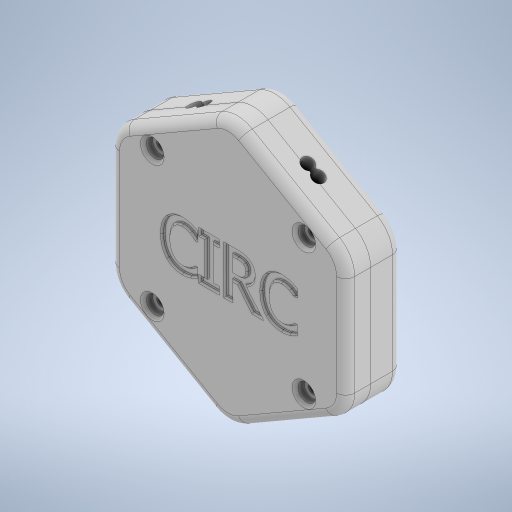
# Autodesk Inventor part: 4-panel splitter
Saved by Autodesk Inventor 2024 (Build 280153020, 153B)
## iProperties
Created: 2023-08-06
Part Number: 4-panel splitter
Material: Generic
Document SubType Name: Modeling
Designer: torban
Density: 1 g/cm^3
Appearance: Default
Author: torban
Autodesk Inventor part; units mm, degrees
(part 1 of 2)
sketch "Sketch2" plane through (0, 0, 0) normal (0, 0, 1) x (1, 0, 0)
  line L0 (0, 0) -> (-18.7, 0)
  line L1 (-18.7, 0) -> (-18.7, 30.4)
  line L2 (-18.7, 30.4) -> (0, 30.4)
  line L3 (0, 30.4) -> (0, 0)
  line L4 (30, 0) -> (48.7, 0)
  line L5 (48.7, 0) -> (48.7, 30.4)
  line L6 (48.7, 30.4) -> (30, 30.4)
  line L7 (30, 30.4) -> (30, 0)
  dimension "d0" = 18.7
  dimension "d1" = 30.4
  dimension "d2" = 30
  dimension "d3" = 30.4
  dimension "d4" = 18.7
  dimension "d5" = 30.4
  constraints: 16 end point, 4 parallel, 2 horizontal, 2 perpendicular
  measures "d0" distance of L1.end L2.end
  measures "d1" distance of L0.end L1.end
  measures "d2" distance between parallel lines of L7 L3
  measures "d3" distance of L4.end L5.end
  measures "d4" distance of L5.end L6.end
  measures "d5" distance between parallel lines of L4 L2
extrude "Extrusion1" add sketch "Sketch2" along normal blind 8.5
sketch "Sketch3" plane through (0, 0, 0) normal (0, 0, -1) x (-1, 0, 0)
  line L0 (-30, 0) -> (-48.7, 0) projected
  line L1 (-48.7, 0) -> (-48.7, 30.4) projected
  line L2 (-48.7, 30.4) -> (-30, 30.4) projected
  line L3 (-30, 30.4) -> (-30, 0) projected
  line L4 (0, 0) -> (0, 30.4) projected
  line L5 (0, 30.4) -> (18.7, 30.4) projected
  line L6 (18.7, 30.4) -> (18.7, 0) projected
  line L7 (18.7, 0) -> (0, 0) projected
  line L8 (-0.2, -0.2) -> (-0.2, 30.6)
  line L9 (-0.2, 30.6) -> (18.9, 30.6)
  line L10 (18.9, 30.6) -> (18.9, -0.2)
  line L11 (18.9, -0.2) -> (-0.2, -0.2)
  line L12 (-48.9, -0.2) -> (-29.8, -0.2)
  line L13 (-29.8, -0.2) -> (-29.8, 30.6)
  line L14 (-29.8, 30.6) -> (-48.9, 30.6)
  line L15 (-48.9, 30.6) -> (-48.9, -0.2)
  line L16 (18.7, 30.4) -> (-48.7, 0) construction
  line L17 (-15, 15.2) -> (-15, 54.3443) construction
  line L18 (-15, 54.3443) -> (18.9, 34.7722)
  line L19 (18.9, 34.7722) -> (18.9, -4.3722)
  line L20 (18.9, -4.3722) -> (-15, -23.9443)
  line L21 (-15, -23.9443) -> (-48.9, -4.3722)
  line L22 (-48.9, -4.3722) -> (-48.9, 34.7722)
  line L23 (-48.9, 34.7722) -> (-15, 54.3443)
  line L24 (-15, -29.7179) -> (23.9, -7.2589)
  line L25 (23.9, -7.2589) -> (23.9, 37.6589)
  line L26 (23.9, 37.6589) -> (-15, 60.1179)
  line L27 (-15, 60.1179) -> (-53.9, 37.6589)
  line L28 (-53.9, 37.6589) -> (-53.9, -7.2589)
  line L29 (-53.9, -7.2589) -> (-15, -29.7179)
  dimension "d14" = 0.2
  dimension "d15" = 0.2
  dimension "d21" = 0
  dimension "d22" = 5
  constraints: 44 end point, 1 coincident, 1 midpoint, 1 vertical, 24 other
  measures "d14" distance between parallel lines of L7 L11
  measures "d15" distance between parallel lines of L0 L12
  measures "d21" distance between parallel lines of L15 L22
  measures "d22" distance between parallel lines of L20 L24
extrude "Extrusion2" add sketch "Sketch3" along normal blind 5 separate body contours L0 L1 L2 L3 | L4 L5 L6 L7 | L11 L19 L20 L21 L22 L12 L13 L14 L23 L18 L9 L8 | L8 L9 L10 L11 | L15 L14 L13 L12 | L29 L28 L27 L26 L25 L24
fillet "Fillet1" radius 10 6 edges at (-23.9, 37.6589, -2.5) (-23.9, -7.2589, -2.5) (15, -29.7179, -2.5) (53.9, -7.2589, -2.5) (53.9, 37.6589, -2.5) (15, 60.1179, -2.5)
sketch "Sketch4" plane through (0, 0, 0) normal (0, 0, 1) x (1, 0, 0)
  line L0 (48.7, 0) -> (30, 0) projected
  line L1 (30, 0) -> (30, 30.4) projected
  line L2 (30, 30.4) -> (48.7, 30.4) projected
  line L3 (48.7, 30.4) -> (48.7, 0) projected
  line L4 (0, 30.4) -> (0, 0) projected
  line L5 (0, 0) -> (-18.7, 0) projected
  line L6 (-18.7, 0) -> (-18.7, 30.4) projected
  line L7 (-18.7, 30.4) -> (0, 30.4) projected
  arc A0 (20, 57.2311) -> (10, 57.2311) centre (15, 48.5708) ccw projected
  line L8 (20, 57.2311) -> (48.9, 40.5457) projected
  arc A1 (53.9, 31.8854) -> (48.9, 40.5457) centre (43.9, 31.8854) ccw projected
  line L9 (53.9, 31.8854) -> (53.9, -1.4854) projected
  arc A2 (48.9, -10.1457) -> (53.9, -1.4854) centre (43.9, -1.4854) ccw projected
  line L10 (48.9, -10.1457) -> (20, -26.8311) projected
  arc A3 (10, -26.8311) -> (20, -26.8311) centre (15, -18.1708) ccw projected
  line L11 (10, -26.8311) -> (-18.9, -10.1457) projected
  arc A4 (-23.9, -1.4854) -> (-18.9, -10.1457) centre (-13.9, -1.4854) ccw projected
  line L12 (-23.9, -1.4854) -> (-23.9, 31.8854) projected
  arc A5 (-18.9, 40.5457) -> (-23.9, 31.8854) centre (-13.9, 31.8854) ccw projected
  line L13 (-18.9, 40.5457) -> (10, 57.2311) projected
  arc A6 (17.5, 52.901) -> (12.5, 52.901) centre (15, 48.5708) ccw
  line L14 (17.5, 52.901) -> (46.4, 36.2155)
  arc A7 (48.9, 31.8854) -> (46.4, 36.2155) centre (43.9, 31.8854) ccw
  line L15 (48.9, 31.8854) -> (48.9, -1.4854)
  arc A8 (46.4, -5.8155) -> (48.9, -1.4854) centre (43.9, -1.4854) ccw
  line L16 (46.4, -5.8155) -> (17.5, -22.501)
  arc A9 (12.5, -22.501) -> (17.5, -22.501) centre (15, -18.1708) ccw
  line L17 (12.5, -22.501) -> (-16.4, -5.8155)
  arc A10 (-18.9, -1.4854) -> (-16.4, -5.8155) centre (-13.9, -1.4854) ccw
  line L18 (-18.9, -1.4854) -> (-18.9, 31.8854)
  arc A11 (-16.4, 36.2155) -> (-18.9, 31.8854) centre (-13.9, 31.8854) ccw
  line L19 (-16.4, 36.2155) -> (12.5, 52.901)
  dimension "d26" = 0.2
  constraints: 12 end point, 12 point on circle, 6 centre point, 11 other
  measures "d26" distance between parallel lines of L6 L18
ref_plane "Work Plane1" through (0, 0, 4.25) normal (0, 0, 1) x (1, 0, 0)
extrude "Extrusion3" add sketch "Sketch4" along normal blind 5.25 contours L8 A1 L9 A2 L10 A3 L11 A4 L12 A5 L13 A0 bodies 2
sketch "Sketch15" plane through (0, 0, 5.25) normal (0, 0, 1) x (1, 0, 0)
  line L0 (48.7, 0) -> (30, 0) projected
  line L1 (30, 0) -> (30, 30.4) projected
  line L2 (30, 30.4) -> (48.7, 30.4) projected
  line L3 (48.7, 30.4) -> (48.7, 0) projected
  line L4 (0, 30.4) -> (0, 0) projected
  line L5 (0, 0) -> (-18.7, 0) projected
  line L6 (-18.7, 0) -> (-18.7, 30.4) projected
  line L7 (-18.7, 30.4) -> (0, 30.4) projected
  arc A0 (48.9, 31.8854) -> (46.4, 36.2155) centre (43.9, 31.8854) ccw projected
  line L8 (46.4, 36.2155) -> (17.5, 52.901) projected
  arc A1 (17.5, 52.901) -> (12.5, 52.901) centre (15, 48.5708) ccw projected
  line L9 (12.5, 52.901) -> (-16.4, 36.2155) projected
  arc A2 (-16.4, 36.2155) -> (-18.9, 31.8854) centre (-13.9, 31.8854) ccw projected
  line L10 (-18.9, 31.8854) -> (-18.9, -1.4854) projected
  arc A3 (-18.9, -1.4854) -> (-16.4, -5.8155) centre (-13.9, -1.4854) ccw projected
  line L11 (-16.4, -5.8155) -> (12.5, -22.501) projected
  arc A4 (12.5, -22.501) -> (17.5, -22.501) centre (15, -18.1708) ccw projected
  line L12 (17.5, -22.501) -> (46.4, -5.8155) projected
  arc A5 (46.4, -5.8155) -> (48.9, -1.4854) centre (43.9, -1.4854) ccw projected
  line L13 (48.9, -1.4854) -> (48.9, 31.8854) projected
  line L14 (20, 57.2311) -> (48.9, 40.5457) projected
  arc A6 (53.9, 31.8854) -> (48.9, 40.5457) centre (43.9, 31.8854) ccw projected
  line L15 (53.9, 31.8854) -> (53.9, -1.4854) projected
  arc A7 (48.9, -10.1457) -> (53.9, -1.4854) centre (43.9, -1.4854) ccw projected
  line L16 (48.9, -10.1457) -> (20, -26.8311) projected
  arc A8 (10, -26.8311) -> (20, -26.8311) centre (15, -18.1708) ccw projected
  line L17 (10, -26.8311) -> (-18.9, -10.1457) projected
  arc A9 (-23.9, -1.4854) -> (-18.9, -10.1457) centre (-13.9, -1.4854) ccw projected
  line L18 (-23.9, -1.4854) -> (-23.9, 31.8854) projected
  arc A10 (-18.9, 40.5457) -> (-23.9, 31.8854) centre (-13.9, 31.8854) ccw projected
  line L19 (-18.9, 40.5457) -> (10, 57.2311) projected
  arc A11 (20, 57.2311) -> (10, 57.2311) centre (15, 48.5708) ccw projected
  line L20 (18.85, 55.2392) -> (47.75, 38.5538)
  arc A12 (51.6, 31.8854) -> (47.75, 38.5538) centre (43.9, 31.8854) ccw
  line L21 (51.6, 31.8854) -> (51.6, -1.4854)
  arc A13 (47.75, -8.1538) -> (51.6, -1.4854) centre (43.9, -1.4854) ccw
  line L22 (47.75, -8.1538) -> (18.85, -24.8392)
  arc A14 (11.15, -24.8392) -> (18.85, -24.8392) centre (15, -18.1708) ccw
  line L23 (11.15, -24.8392) -> (-17.75, -8.1538)
  arc A15 (-21.6, -1.4854) -> (-17.75, -8.1538) centre (-13.9, -1.4854) ccw
  line L24 (-21.6, -1.4854) -> (-21.6, 31.8854)
  arc A16 (-17.75, 38.5538) -> (-21.6, 31.8854) centre (-13.9, 31.8854) ccw
  line L25 (-17.75, 38.5538) -> (11.15, 55.2392)
  arc A17 (18.85, 55.2392) -> (11.15, 55.2392) centre (15, 48.5708) ccw
  dimension "d89" = 2.7
  constraints: 12 end point, 12 point on circle, 6 centre point, 11 other
  measures "d89" distance between parallel lines of L8 L20
extrude "Extrusion13" cut sketch "Sketch15" against normal blind 2 contours L20 A12 L21 A13 L22 A14 L23 A15 L24 A16 L25 A17 bodies 2
sketch "Sketch16" plane through (0, 0, 3.25) normal (0, 0, 1) x (1, 0, 0)
  line L0 (48.7, 0) -> (30, 0) projected
  line L1 (30, 0) -> (30, 30.4) projected
  line L2 (30, 30.4) -> (48.7, 30.4) projected
  line L3 (48.7, 30.4) -> (48.7, 0) projected
  line L4 (0, 30.4) -> (0, 0) projected
  line L5 (0, 0) -> (-18.7, 0) projected
  line L6 (-18.7, 0) -> (-18.7, 30.4) projected
  line L7 (-18.7, 30.4) -> (0, 30.4) projected
  arc A0 (-21.6, -1.4854) -> (-17.75, -8.1538) centre (-13.9, -1.4854) ccw projected
  line L8 (-17.75, -8.1538) -> (11.15, -24.8392) projected
  arc A1 (11.15, -24.8392) -> (18.85, -24.8392) centre (15, -18.1708) ccw projected
  line L9 (18.85, -24.8392) -> (47.75, -8.1538) projected
  arc A2 (47.75, -8.1538) -> (51.6, -1.4854) centre (43.9, -1.4854) ccw projected
  line L10 (51.6, -1.4854) -> (51.6, 31.8854) projected
  arc A3 (51.6, 31.8854) -> (47.75, 38.5538) centre (43.9, 31.8854) ccw projected
  line L11 (47.75, 38.5538) -> (18.85, 55.2392) projected
  arc A4 (18.85, 55.2392) -> (11.15, 55.2392) centre (15, 48.5708) ccw projected
  line L12 (11.15, 55.2392) -> (-17.75, 38.5538) projected
  arc A5 (-17.75, 38.5538) -> (-21.6, 31.8854) centre (-13.9, 31.8854) ccw projected
  line L13 (-21.6, 31.8854) -> (-21.6, -1.4854) projected
  line L14 (48.9, -1.4854) -> (48.9, 31.8854) projected
  arc A6 (48.9, 31.8854) -> (46.4, 36.2155) centre (43.9, 31.8854) ccw projected
  line L15 (46.4, 36.2155) -> (17.5, 52.901) projected
  arc A7 (17.5, 52.901) -> (12.5, 52.901) centre (15, 48.5708) ccw projected
  line L16 (12.5, 52.901) -> (-16.4, 36.2155) projected
  arc A8 (-16.4, 36.2155) -> (-18.9, 31.8854) centre (-13.9, 31.8854) ccw projected
  line L17 (-18.9, 31.8854) -> (-18.9, -1.4854) projected
  arc A9 (-18.9, -1.4854) -> (-16.4, -5.8155) centre (-13.9, -1.4854) ccw projected
  line L18 (-16.4, -5.8155) -> (12.5, -22.501) projected
  arc A10 (12.5, -22.501) -> (17.5, -22.501) centre (15, -18.1708) ccw projected
  line L19 (17.5, -22.501) -> (46.4, -5.8155) projected
  arc A11 (46.4, -5.8155) -> (48.9, -1.4854) centre (43.9, -1.4854) ccw projected
  arc A12 (20, 57.2311) -> (10, 57.2311) centre (15, 48.5708) ccw projected
  line L20 (20, 57.2311) -> (48.9, 40.5457) projected
  arc A13 (53.9, 31.8854) -> (48.9, 40.5457) centre (43.9, 31.8854) ccw projected
  line L21 (53.9, 31.8854) -> (53.9, -1.4854) projected
  arc A14 (48.9, -10.1457) -> (53.9, -1.4854) centre (43.9, -1.4854) ccw projected
  line L22 (48.9, -10.1457) -> (20, -26.8311) projected
  arc A15 (10, -26.8311) -> (20, -26.8311) centre (15, -18.1708) ccw projected
  line L23 (10, -26.8311) -> (-18.9, -10.1457) projected
  arc A16 (-23.9, -1.4854) -> (-18.9, -10.1457) centre (-13.9, -1.4854) ccw projected
  line L24 (-23.9, -1.4854) -> (-23.9, 31.8854) projected
  arc A17 (-18.9, 40.5457) -> (-23.9, 31.8854) centre (-13.9, 31.8854) ccw projected
  line L25 (-18.9, 40.5457) -> (10, 57.2311) projected
  line L26 (11.35, -24.4928) -> (-17.55, -7.8074)
  arc A18 (-21.2, -1.4854) -> (-17.55, -7.8074) centre (-13.9, -1.4854) ccw
  line L27 (-21.2, -1.4854) -> (-21.2, 31.8854)
  arc A19 (-17.55, 38.2074) -> (-21.2, 31.8854) centre (-13.9, 31.8854) ccw
  line L28 (-17.55, 38.2074) -> (11.35, 54.8928)
  arc A20 (18.65, 54.8928) -> (11.35, 54.8928) centre (15, 48.5708) ccw
  line L29 (18.65, 54.8928) -> (47.55, 38.2074)
  arc A21 (51.2, 31.8854) -> (47.55, 38.2074) centre (43.9, 31.8854) ccw
  line L30 (51.2, 31.8854) -> (51.2, -1.4854)
  arc A22 (47.55, -7.8074) -> (51.2, -1.4854) centre (43.9, -1.4854) ccw
  line L31 (47.55, -7.8074) -> (18.65, -24.4928)
  arc A23 (11.35, -24.4928) -> (18.65, -24.4928) centre (15, -18.1708) ccw
  dimension "d92" = 2.3
  constraints: 12 end point, 12 point on circle, 6 centre point, 11 other
  measures "d92" distance between parallel lines of L18 L26
extrude "Extrusion14" add sketch "Sketch16" along normal blind 2 separate body contours L26 A18 L27 A19 L28 A20 L29 A21 L30 A22 L31 A23
sketch "Sketch17" plane through (0, 0, 5.25) normal (0, 0, 1) x (1, 0, 0)
  line L0 (48.7, 0) -> (30, 0) projected
  line L1 (30, 0) -> (30, 30.4) projected
  line L2 (30, 30.4) -> (48.7, 30.4) projected
  line L3 (48.7, 30.4) -> (48.7, 0) projected
  line L4 (0, 30.4) -> (0, 0) projected
  line L5 (0, 0) -> (-18.7, 0) projected
  line L6 (-18.7, 0) -> (-18.7, 30.4) projected
  line L7 (-18.7, 30.4) -> (0, 30.4) projected
  arc A0 (-21.6, -1.4854) -> (-17.75, -8.1538) centre (-13.9, -1.4854) ccw projected
  line L8 (-17.75, -8.1538) -> (11.15, -24.8392) projected
  arc A1 (11.15, -24.8392) -> (18.85, -24.8392) centre (15, -18.1708) ccw projected
  line L9 (18.85, -24.8392) -> (47.75, -8.1538) projected
  arc A2 (47.75, -8.1538) -> (51.6, -1.4854) centre (43.9, -1.4854) ccw projected
  line L10 (51.6, -1.4854) -> (51.6, 31.8854) projected
  arc A3 (51.6, 31.8854) -> (47.75, 38.5538) centre (43.9, 31.8854) ccw projected
  line L11 (47.75, 38.5538) -> (18.85, 55.2392) projected
  arc A4 (18.85, 55.2392) -> (11.15, 55.2392) centre (15, 48.5708) ccw projected
  line L12 (11.15, 55.2392) -> (-17.75, 38.5538) projected
  arc A5 (-17.75, 38.5538) -> (-21.6, 31.8854) centre (-13.9, 31.8854) ccw projected
  line L13 (-21.6, 31.8854) -> (-21.6, -1.4854) projected
  line L14 (20, 57.2311) -> (48.9, 40.5457) projected
  arc A6 (53.9, 31.8854) -> (48.9, 40.5457) centre (43.9, 31.8854) ccw projected
  line L15 (53.9, 31.8854) -> (53.9, -1.4854) projected
  arc A7 (48.9, -10.1457) -> (53.9, -1.4854) centre (43.9, -1.4854) ccw projected
  line L16 (48.9, -10.1457) -> (20, -26.8311) projected
  arc A8 (10, -26.8311) -> (20, -26.8311) centre (15, -18.1708) ccw projected
  line L17 (10, -26.8311) -> (-18.9, -10.1457) projected
  arc A9 (-23.9, -1.4854) -> (-18.9, -10.1457) centre (-13.9, -1.4854) ccw projected
  line L18 (-23.9, -1.4854) -> (-23.9, 31.8854) projected
  arc A10 (-18.9, 40.5457) -> (-23.9, 31.8854) centre (-13.9, 31.8854) ccw projected
  line L19 (-18.9, 40.5457) -> (10, 57.2311) projected
  arc A11 (20, 57.2311) -> (10, 57.2311) centre (15, 48.5708) ccw projected
  line L20 (48.9, -1.4854) -> (48.9, 31.8854) projected
  arc A12 (48.9, 31.8854) -> (46.4, 36.2155) centre (43.9, 31.8854) ccw projected
  line L21 (46.4, 36.2155) -> (17.5, 52.901) projected
  arc A13 (17.5, 52.901) -> (12.5, 52.901) centre (15, 48.5708) ccw projected
  line L22 (12.5, 52.901) -> (-16.4, 36.2155) projected
  arc A14 (-16.4, 36.2155) -> (-18.9, 31.8854) centre (-13.9, 31.8854) ccw projected
  line L23 (-18.9, 31.8854) -> (-18.9, -1.4854) projected
  arc A15 (-18.9, -1.4854) -> (-16.4, -5.8155) centre (-13.9, -1.4854) ccw projected
  line L24 (-16.4, -5.8155) -> (12.5, -22.501) projected
  arc A16 (12.5, -22.501) -> (17.5, -22.501) centre (15, -18.1708) ccw projected
  line L25 (17.5, -22.501) -> (46.4, -5.8155) projected
  arc A17 (46.4, -5.8155) -> (48.9, -1.4854) centre (43.9, -1.4854) ccw projected
  arc A18 (47.55, -7.8074) -> (51.2, -1.4854) centre (43.9, -1.4854) ccw projected
  line L26 (47.55, -7.8074) -> (18.65, -24.4928) projected
  arc A19 (11.35, -24.4928) -> (18.65, -24.4928) centre (15, -18.1708) ccw projected
  line L27 (11.35, -24.4928) -> (-17.55, -7.8074) projected
  arc A20 (-21.2, -1.4854) -> (-17.55, -7.8074) centre (-13.9, -1.4854) ccw projected
  line L28 (-21.2, -1.4854) -> (-21.2, 31.8854) projected
  arc A21 (-17.55, 38.2074) -> (-21.2, 31.8854) centre (-13.9, 31.8854) ccw projected
  line L29 (-17.55, 38.2074) -> (11.35, 54.8928) projected
  arc A22 (18.65, 54.8928) -> (11.35, 54.8928) centre (15, 48.5708) ccw projected
  line L30 (18.65, 54.8928) -> (47.55, 38.2074) projected
  arc A23 (51.2, 31.8854) -> (47.55, 38.2074) centre (43.9, 31.8854) ccw projected
  line L31 (51.2, 31.8854) -> (51.2, -1.4854) projected
extrude "Extrusion15" add sketch "Sketch17" along normal up to surface (3.25 mm away) contours L13 A5 L12 A4 L11 A3 L10 A2 L9 A1 L8 A0 | L14 A6 L15 A7 L16 A8 L17 A9 L18 A10 L19 A11 | L26 A19 L27 A20 L28 A21 L29 A22 L30 A23 L31 A18 bodies 3
sketch "Sketch18" plane through (10, 57.2311, 5.25) normal (-0.5, 0.8660254, 0) x (0.8660254, 0.5, 0)
  line L0 (0, 0) -> (-33.3708, 0) projected
  line L1 (-33.3708, 2) -> (0, 2) projected
  line L2 (0, 5.25) -> (-33.3708, 5.25) projected
  line L3 (0, -3.25) -> (-33.3708, -3.25) projected
  line L4 (0, 10.25) -> (0, 0) projected
  line L5 (0, 0) -> (0, 2)
  line L6 (0, 1) -> (-33.3708, 1)
  circle A0 centre (-2, 1) radius 2
  circle A1 centre (-6, 1) radius 2
  circle A2 centre (-14, 1) radius 2
  circle A3 centre (-18, 1) radius 2
  point P0 (-37.2758, 5.25)
  point P1 (-4, 1)
  point P2 (-16, 1)
  dimension "d97" = 4
  dimension "d98" = 4
  dimension "d99" = 4
  dimension "d100" = 4
  dimension "d101" = 4
  dimension "d102" = 8
  dimension "d103" = 4
  dimension "d104" = 2
  constraints: 4 centre point, 4 end point, 4 point on line, 1 horizontal, 1 midpoint, 1 perpendicular
  measures "d97" diameter of A0
  measures "d98" diameter of A1
  measures "d99" diameter of A2
  measures "d100" diameter of A3
  measures "d101" distance of A1.centre A0.centre
  measures "d102" distance of A2.centre A1.centre
  measures "d103" distance of A2.centre A3.centre
  measures "d104" distance of L6.start A0.centre
extrude "Extrusion16" cut sketch "Sketch18" against normal blind 5 contours A2 L0 L6 | L6 A2 L1 | A2 L0 | A3 L0 L6 | L6 A3 L1 | L1 A2 | L1 A3 | A3 L0 bodies 2 3
ref_plane "Work Plane7" through (15, 0, 0) normal (1, 0, 0) x (0, 0, -1)
mirror "Mirror5" about plane through (15, 0, 0) normal (1, 0, 0) of "Extrusion16" bodies 2 3
ref_plane "Work Plane9" through (-18.7, -1, 0) normal (0, -1, 0) x (1, 0, 0)
sketch "Sketch19" plane through (-18.7, -1, 0) normal (0, -1, 0) x (1, 0, 0)
  line L0 (28.7, -5) -> (28.7, 5.25) projected
  line L1 (38.7, -5) -> (38.7, 5.25) projected
  line L2 (29.4679, 4.25) -> (38.7, 4.25)
  circle A0 centre (35.7, 4.25) radius 2
  circle A1 centre (31.7, 4.25) radius 2
  point P0 (18.7, 0)
  point P1 (33.7, 4.25)
  dimension "d108" = 4
  dimension "d109" = 4
  dimension "d110" = 4
  dimension "d111" = 3
  dimension "d112" = 3
  constraints: 3 point on line, 2 centre point, 2 end point, 1 horizontal
  measures "d108" diameter of A0
  measures "d109" diameter of A1
  measures "d110" distance of A0.centre A1.centre
  measures "d111" distance from line of L1 A0.centre
  measures "d112" distance from line of L0 A1.centre
extrude "Extrusion17" cut sketch "Sketch19" along normal through all bodies 1 3 2
sketch "Sketch20" plane through (0, 0, 0) normal (0, 0, 1) x (1, 0, 0)
  line L0 (0, 30.4) -> (0, 0) projected
  line L1 (0, 0) -> (-18.7, 0) projected
  line L2 (-18.7, 0) -> (-18.7, 30.4) projected
  line L3 (-18.7, 30.4) -> (0, 30.4) projected
  line L4 (48.7, 0) -> (30, 0) projected
  line L5 (30, 0) -> (30, 30.4) projected
  line L6 (30, 30.4) -> (48.7, 30.4) projected
  line L7 (48.7, 30.4) -> (48.7, 0) projected
  line L8 (-18.9, 40.5457) -> (10, 57.2311) projected
  arc A0 (20, 57.2311) -> (10, 57.2311) centre (15, 48.5708) ccw projected
  line L9 (20, 57.2311) -> (48.9, 40.5457) projected
  arc A1 (53.9, 31.8854) -> (48.9, 40.5457) centre (43.9, 31.8854) ccw projected
  line L10 (53.9, 31.8854) -> (53.9, -1.4854) projected
  arc A2 (48.9, -10.1457) -> (53.9, -1.4854) centre (43.9, -1.4854) ccw projected
  line L11 (48.9, -10.1457) -> (20, -26.8311) projected
  arc A3 (10, -26.8311) -> (20, -26.8311) centre (15, -18.1708) ccw projected
  line L12 (10, -26.8311) -> (-18.9, -10.1457) projected
  arc A4 (-23.9, -1.4854) -> (-18.9, -10.1457) centre (-13.9, -1.4854) ccw projected
  line L13 (-23.9, -1.4854) -> (-23.9, 31.8854) projected
  arc A5 (-18.9, 40.5457) -> (-23.9, 31.8854) centre (-13.9, 31.8854) ccw projected
  line L14 (12.5, 52.901) -> (-16.4, 36.2155) projected
  arc A6 (-16.4, 36.2155) -> (-18.9, 31.8854) centre (-13.9, 31.8854) ccw projected
  line L15 (-18.9, 31.8854) -> (-18.9, -1.4854) projected
  arc A7 (-18.9, -1.4854) -> (-16.4, -5.8155) centre (-13.9, -1.4854) ccw projected
  line L16 (-16.4, -5.8155) -> (12.5, -22.501) projected
  arc A8 (12.5, -22.501) -> (17.5, -22.501) centre (15, -18.1708) ccw projected
  line L17 (17.5, -22.501) -> (46.4, -5.8155) projected
  arc A9 (46.4, -5.8155) -> (48.9, -1.4854) centre (43.9, -1.4854) ccw projected
  line L18 (48.9, -1.4854) -> (48.9, 31.8854) projected
  arc A10 (48.9, 31.8854) -> (46.4, 36.2155) centre (43.9, 31.8854) ccw projected
  line L19 (46.4, 36.2155) -> (17.5, 52.901) projected
  arc A11 (17.5, 52.901) -> (12.5, 52.901) centre (15, 48.5708) ccw projected
  line L20 (0.2, -0.2) -> (0.2, 30.6)
  line L21 (0.2, 30.6) -> (-18.9, 30.6)
  line L22 (-18.9, 30.6) -> (-18.9, -0.2)
  line L23 (-18.9, -0.2) -> (0.2, -0.2)
  line L24 (29.8, 30.6) -> (29.8, -0.2)
  line L25 (29.8, -0.2) -> (48.9, -0.2)
  line L26 (48.9, -0.2) -> (48.9, 30.6)
  line L27 (48.9, 30.6) -> (29.8, 30.6)
  line L28 (29.8, -0.2) -> (29.8, 0.8)
  line L29 (29.8, 0.8) -> (28.8, 0.8)
  line L30 (0.2, -0.2) -> (0.2, 0.8)
  line L31 (0.2, 0.8) -> (1.2, 0.8)
  line L32 (0.2, 30.6) -> (0.2, 29.6)
  line L33 (0.2, 29.6) -> (1.2, 29.6)
  line L34 (29.8, 30.6) -> (29.8, 29.6)
  line L35 (29.8, 29.6) -> (28.8, 29.6)
  line L36 (-1.5885, 44.767) -> (-4.5885, 43.0349) projected
  line L37 (-1.3564, 44.901) -> (-4.8205, 42.901) projected
  line L38 (34.5885, 43.0349) -> (31.5885, 44.767) projected
  line L39 (34.8205, 42.901) -> (31.3564, 44.901) projected
  line L40 (-4.8205, 42.901) -> (1.2, 29.6)
  line L41 (28.8, 29.6) -> (34.8205, 42.901)
  line L42 (1.2, 0.8) -> (-4.8205, -12.501)
  line L43 (-16.4, -5.8155) -> (12.5, -22.501) projected
  line L44 (28.8, 0.8) -> (34.8205, -12.501)
  point P0 (-18.9, -0.2)
  dimension "d115" = 0.2
  dimension "d116" = 0.2
  dimension "d117" = 1
  dimension "d118" = 1
  dimension "d119" = 1
  dimension "d120" = 1
  dimension "d121" = 1
  dimension "d122" = 1
  dimension "d123" = 1
  dimension "d124" = 1
  dimension "d125" = 65.647
  dimension "d126" = 65.647
  dimension "d127" = 65.647
  dimension "d128" = 65.647
  constraints: 40 end point, 6 point on line, 4 perpendicular, 6 other
  measures "d115" distance between parallel lines of L0 L20
  measures "d116" distance between parallel lines of L5 L24
  measures "d117" distance of L24.end L28.end
  measures "d118" distance of L28.end L29.end
  measures "d119" distance of L20.start L30.end
  measures "d120" distance of L30.end L31.end
  measures "d121" distance of L20.end L32.end
  measures "d122" distance of L32.end L33.end
  measures "d123" distance of L24.start L34.end
  measures "d124" distance of L34.end L35.end
  measures "d125" angle of L21 L40
  measures "d126" angle of L41 L27
  measures "d127" angle of L44 L25
  measures "d128" angle of L23 L42
extrude "Extrusion18" add sketch "Sketch20" along normal up to surface (3.25 mm away) contours L40 L33 L20 L21 L15 A6 L14 | L19 A10 L18 L27 L24 L35 L41 | L31 L42 L16 A7 L15 L23 L20 | L24 L25 L18 A9 L17 L44 L29 bodies 2
sketch "Sketch21" plane through (0, 0, 3.25) normal (0, 0, 1) x (1, 0, 0)
  line L0 (0, 30.4) -> (0, 0) projected
  line L1 (0, 0) -> (-18.7, 0) projected
  line L2 (-18.7, 0) -> (-18.7, 30.4) projected
  line L3 (-18.7, 30.4) -> (0, 30.4) projected
  line L4 (48.7, 0) -> (30, 0) projected
  line L5 (30, 0) -> (30, 30.4) projected
  line L6 (30, 30.4) -> (48.7, 30.4) projected
  line L7 (48.7, 30.4) -> (48.7, 0) projected
  line L8 (18.7321, -27.4483) -> (18.7321, -24.906) projected
  line L9 (18.7321, -24.906) -> (18.7321, -21.7896) projected
  line L10 (18.7321, -21.7896) -> (34.8205, -12.501) projected
  line L11 (34.8205, -12.501) -> (28.8, 0.8) projected
  line L12 (28.8, 0.8) -> (29.8, 0.8) projected
  line L13 (29.8, 0.8) -> (29.8, -0.2) projected
  line L14 (29.8, -0.2) -> (48.9, -0.2) projected
  line L15 (48.9, -0.2) -> (48.9, 30.6) projected
  line L16 (48.9, 30.6) -> (29.8, 30.6) projected
  line L17 (29.8, 30.6) -> (29.8, 29.6) projected
  line L18 (29.8, 29.6) -> (28.8, 29.6) projected
  line L19 (28.8, 29.6) -> (34.8205, 42.901) projected
  line L20 (34.8205, 42.901) -> (34.5885, 43.0349) projected
  line L21 (34.5885, 43.0349) -> (35.9385, 45.3732) projected
  line L22 (35.9385, 45.3732) -> (37.0885, 47.3651) projected
  line L23 (37.0885, 47.3651) -> (48.9, 40.5457) projected
  arc A0 (53.9, 31.8854) -> (48.9, 40.5457) centre (43.9, 31.8854) ccw projected
  line L24 (53.9, 31.8854) -> (53.9, -1.4854) projected
  arc A1 (48.9, -10.1457) -> (53.9, -1.4854) centre (43.9, -1.4854) ccw projected
  line L25 (48.9, -10.1457) -> (20, -26.8311) projected
  arc A2 (18.7321, -27.4483) -> (20, -26.8311) centre (15, -18.1708) ccw projected
  arc A3 (18.7321, -24.906) -> (18.85, -24.8392) centre (15, -18.1708) ccw projected
  line L26 (47.75, -8.1538) -> (18.85, -24.8392) projected
  arc A4 (47.75, -8.1538) -> (51.6, -1.4854) centre (43.9, -1.4854) ccw projected
  line L27 (51.6, 31.8854) -> (51.6, -1.4854) projected
  arc A5 (51.6, 31.8854) -> (47.75, 38.5538) centre (43.9, 31.8854) ccw projected
  line L28 (35.9385, 45.3732) -> (47.75, 38.5538) projected
  line L29 (15.2679, -23.1637) -> (15.2679, -25.8662) projected
  line L30 (15.2679, -25.8662) -> (15.2679, -28.1673) projected
  arc A6 (14.7321, -28.1673) -> (15.2679, -28.1673) centre (15, -18.1708) ccw projected
  line L31 (14.7321, -28.1673) -> (14.7321, -25.8662) projected
  arc A7 (14.7321, -25.8662) -> (15.2679, -25.8662) centre (15, -18.1708) ccw projected
  arc A8 (14.7321, -23.1637) -> (15.2679, -23.1637) centre (15, -18.1708) ccw projected
  line L32 (14.7321, -25.8662) -> (14.7321, -23.1637) projected
  line L33 (11.15, -24.8392) -> (-17.75, -8.1538) projected
  arc A9 (11.15, -24.8392) -> (11.2679, -24.906) centre (15, -18.1708) ccw projected
  line L34 (11.2679, -24.906) -> (11.2679, -27.4483) projected
  arc A10 (10, -26.8311) -> (11.2679, -27.4483) centre (15, -18.1708) ccw projected
  line L35 (10, -26.8311) -> (-18.9, -10.1457) projected
  arc A11 (-23.9, -1.4854) -> (-18.9, -10.1457) centre (-13.9, -1.4854) ccw projected
  line L36 (-23.9, -1.4854) -> (-23.9, 31.8854) projected
  arc A12 (-18.9, 40.5457) -> (-23.9, 31.8854) centre (-13.9, 31.8854) ccw projected
  line L37 (-18.9, 40.5457) -> (-7.0885, 47.3651) projected
  line L38 (-7.0885, 47.3651) -> (-5.9385, 45.3732) projected
  line L39 (-5.9385, 45.3732) -> (-4.5885, 43.0349) projected
  line L40 (-4.8205, 42.901) -> (1.2, 29.6) projected
  line L41 (1.2, 29.6) -> (0.2, 29.6) projected
  line L42 (0.2, 29.6) -> (0.2, 30.6) projected
  line L43 (0.2, 30.6) -> (-18.9, 30.6) projected
  line L44 (-18.9, 30.6) -> (-18.9, -0.2) projected
  line L45 (-18.9, -0.2) -> (0.2, -0.2) projected
  line L46 (0.2, -0.2) -> (0.2, 0.8) projected
  line L47 (0.2, 0.8) -> (1.2, 0.8) projected
  line L48 (1.2, 0.8) -> (-4.8205, -12.501) projected
  line L49 (-4.8205, -12.501) -> (11.2679, -21.7896) projected
  line L50 (11.2679, -21.7896) -> (11.2679, -24.906) projected
  arc A13 (-21.6, -1.4854) -> (-17.75, -8.1538) centre (-13.9, -1.4854) ccw projected
  line L51 (-21.6, -1.4854) -> (-21.6, 31.8854) projected
  arc A14 (-17.75, 38.5538) -> (-21.6, 31.8854) centre (-13.9, 31.8854) ccw projected
  line L52 (-17.75, 38.5538) -> (-5.9385, 45.3732) projected
  line L53 (34.0885, 49.0971) -> (32.9385, 47.1053) projected
  line L54 (32.9385, 47.1053) -> (31.5885, 44.767) projected
  line L55 (31.1244, 45.0349) -> (32.4744, 47.3732) projected
  line L56 (33.6244, 49.3651) -> (34.0885, 49.0971) projected
  line L57 (32.4744, 47.3732) -> (33.6244, 49.3651) projected
  line L58 (30.6244, 51.0971) -> (29.4744, 49.1053) projected
  line L59 (29.4744, 49.1053) -> (28.1244, 46.767) projected
  line L60 (28.1244, 46.767) -> (17.5, 52.901) projected
  arc A15 (17.5, 52.901) -> (12.5, 52.901) centre (15, 48.5708) ccw projected
  line L61 (12.5, 52.901) -> (1.8756, 46.767) projected
  line L62 (-0.6244, 51.0971) -> (10, 57.2311) projected
  arc A16 (20, 57.2311) -> (10, 57.2311) centre (15, 48.5708) ccw projected
  line L63 (20, 57.2311) -> (30.6244, 51.0971) projected
  line L64 (29.4744, 49.1053) -> (18.85, 55.2392) projected
  arc A17 (18.85, 55.2392) -> (11.15, 55.2392) centre (15, 48.5708) ccw projected
  line L65 (1.8756, 46.767) -> (0.5256, 49.1053) projected
  line L66 (0.5256, 49.1053) -> (-0.6244, 51.0971) projected
  line L67 (-3.6244, 49.3651) -> (-2.4744, 47.3732) projected
  line L68 (-2.4744, 47.3732) -> (-1.1244, 45.0349) projected
  line L69 (-1.5885, 44.767) -> (-2.9385, 47.1053) projected
  line L70 (-4.0885, 49.0971) -> (-3.6244, 49.3651) projected
  line L71 (-2.9385, 47.1053) -> (-4.0885, 49.0971) projected
  line L72 (11.2679, -21.7896) -> (11.2679, -24.4455) projected
  line L73 (11.2679, -24.4455) -> (-17.55, -7.8074) projected
  arc A18 (-21.2, -1.4854) -> (-17.55, -7.8074) centre (-13.9, -1.4854) ccw projected
  line L74 (-21.2, -1.4854) -> (-21.2, 31.8854) projected
  arc A19 (-17.55, 38.2074) -> (-21.2, 31.8854) centre (-13.9, 31.8854) ccw projected
  line L75 (-5.7385, 45.0268) -> (-4.5885, 43.0349) projected
  arc A20 (-16.4, 36.2155) -> (-18.9, 31.8854) centre (-13.9, 31.8854) ccw projected
  line L76 (-18.9, 31.8854) -> (-18.9, -1.4854) projected
  arc A21 (-18.9, -1.4854) -> (-16.4, -5.8155) centre (-13.9, -1.4854) ccw projected
  line L77 (-16.4, -5.8155) -> (11.2679, -21.7896) projected
  line L78 (18.7321, -24.4455) -> (18.7321, -21.7896) projected
  line L79 (18.7321, -21.7896) -> (46.4, -5.8155) projected
  arc A22 (46.4, -5.8155) -> (48.9, -1.4854) centre (43.9, -1.4854) ccw projected
  line L80 (48.9, -1.4854) -> (48.9, 31.8854) projected
  arc A23 (48.9, 31.8854) -> (46.4, 36.2155) centre (43.9, 31.8854) ccw projected
  line L81 (46.4, 36.2155) -> (34.5885, 43.0349) projected
  line L82 (34.5885, 43.0349) -> (35.7385, 45.0268) projected
  line L83 (35.7385, 45.0268) -> (47.55, 38.2074) projected
  arc A24 (51.2, 31.8854) -> (47.55, 38.2074) centre (43.9, 31.8854) ccw projected
  line L84 (51.2, 31.8854) -> (51.2, -1.4854) projected
  arc A25 (47.55, -7.8074) -> (51.2, -1.4854) centre (43.9, -1.4854) ccw projected
  line L85 (47.55, -7.8074) -> (18.7321, -24.4455) projected
  line L86 (14.7321, -25.4659) -> (14.7321, -23.1637) projected
  arc A26 (14.7321, -23.1637) -> (15.2679, -23.1637) centre (15, -18.1708) ccw projected
  line L87 (15.2679, -23.1637) -> (15.2679, -25.4659) projected
  arc A27 (14.7321, -25.4659) -> (15.2679, -25.4659) centre (15, -18.1708) ccw projected
  line L88 (32.7385, 46.7589) -> (31.5885, 44.767) projected
  line L89 (31.1244, 45.0349) -> (32.2744, 47.0268) projected
  line L90 (29.2744, 48.7589) -> (28.1244, 46.767) projected
  line L91 (28.1244, 46.767) -> (17.5, 52.901) projected
  arc A28 (17.5, 52.901) -> (12.5, 52.901) centre (15, 48.5708) ccw projected
  line L92 (12.5, 52.901) -> (1.8756, 46.767) projected
  line L93 (0.7256, 48.7589) -> (11.35, 54.8928) projected
  arc A29 (18.65, 54.8928) -> (11.35, 54.8928) centre (15, 48.5708) ccw projected
  line L94 (18.65, 54.8928) -> (29.2744, 48.7589) projected
  line L95 (1.8756, 46.767) -> (0.7256, 48.7589) projected
  line L96 (-1.5885, 44.767) -> (-2.7385, 46.7589) projected
  line L97 (-2.2744, 47.0268) -> (-1.1244, 45.0349) projected
  line L98 (-4.5885, 43.0349) -> (-4.8205, 42.901) projected
  line L99 (11.15, 55.2392) -> (0.5256, 49.1053) projected
  line L100 (31.5885, 44.767) -> (31.1244, 45.0349) projected
  line L101 (32.4744, 47.3732) -> (32.9385, 47.1053) projected
  line L102 (-1.1244, 45.0349) -> (-1.5885, 44.767) projected
  line L103 (-2.9385, 47.1053) -> (-2.4744, 47.3732) projected
  line L104 (-17.55, 38.2074) -> (-5.7385, 45.0268) projected
  line L105 (-4.5885, 43.0349) -> (-16.4, 36.2155) projected
  line L106 (31.5885, 44.767) -> (31.1244, 45.0349) projected
  line L107 (32.2744, 47.0268) -> (32.7385, 46.7589) projected
  line L108 (-2.7385, 46.7589) -> (-2.2744, 47.0268) projected
  line L109 (-1.1244, 45.0349) -> (-1.5885, 44.767) projected
extrude "Extrusion19" add sketch "Sketch21" along normal up to surface (5.25 mm away) contours L11 L12 L13 L14 L80 A22 L79 | L16 L17 L18 L19 L81 A23 L80 | L77 A21 L76 L45 L46 L47 L48 | L40 L41 L42 L43 L76 A20 L105 bodies 3
sketch "Sketch22" plane through (15, -18.1708, 8.5) normal (0, 0, 1) x (1, 0, 0)
  line L0 (-15, 48.5708) -> (-15, 18.1708) projected
  line L1 (-15, 18.1708) -> (-33.7, 18.1708) projected
  line L2 (-33.7, 18.1708) -> (-33.7, 48.5708) projected
  line L3 (-33.7, 48.5708) -> (-15, 48.5708) projected
  line L4 (33.7, 18.1708) -> (15, 18.1708) projected
  line L5 (15, 18.1708) -> (15, 48.5708) projected
  line L6 (15, 48.5708) -> (33.7, 48.5708) projected
  line L7 (33.7, 48.5708) -> (33.7, 18.1708) projected
  line L8 (-14.8, 48.7708) -> (-33.9, 48.7708) projected
  line L9 (-33.9, 48.7708) -> (-33.9, 17.9708) projected
  line L10 (-33.9, 17.9708) -> (-14.8, 17.9708) projected
  line L11 (-14.8, 17.9708) -> (-14.8, 18.9708) projected
  line L12 (-14.8, 18.9708) -> (-13.8, 18.9708) projected
  line L13 (-13.8, 18.9708) -> (-19.8205, 5.6699) projected
  line L14 (-19.8205, 5.6699) -> (-2.5, -4.3301) projected
  arc A0 (-2.5, -4.3301) -> (2.5, -4.3301) centre (0, 0) ccw projected
  line L15 (2.5, -4.3301) -> (19.8205, 5.6699) projected
  line L16 (19.8205, 5.6699) -> (13.8, 18.9708) projected
  line L17 (13.8, 18.9708) -> (14.8, 18.9708) projected
  line L18 (14.8, 18.9708) -> (14.8, 17.9708) projected
  line L19 (14.8, 17.9708) -> (33.9, 17.9708) projected
  line L20 (33.9, 17.9708) -> (33.9, 48.7708) projected
  line L21 (33.9, 48.7708) -> (14.8, 48.7708) projected
  line L22 (14.8, 48.7708) -> (14.8, 47.7708) projected
  line L23 (14.8, 47.7708) -> (13.8, 47.7708) projected
  line L24 (13.8, 47.7708) -> (19.8205, 61.0718) projected
  line L25 (19.8205, 61.0718) -> (2.5, 71.0718) projected
  arc A1 (2.5, 71.0718) -> (-2.5, 71.0718) centre (0, 66.7417) ccw projected
  line L26 (-2.5, 71.0718) -> (-19.8205, 61.0718) projected
  line L27 (-19.8205, 61.0718) -> (-13.8, 47.7708) projected
  line L28 (-13.8, 47.7708) -> (-14.8, 47.7708) projected
  line L29 (-14.8, 47.7708) -> (-14.8, 48.7708) projected
  arc A2 (33.9, 8.0252) -> (38.9, 16.6854) centre (28.9, 16.6854) ccw projected
  line L30 (33.9, 8.0252) -> (5, -8.6603) projected
  arc A3 (-5, -8.6603) -> (5, -8.6603) centre (0, 0) ccw projected
  line L31 (-5, -8.6603) -> (-33.9, 8.0252) projected
  arc A4 (-38.9, 16.6854) -> (-33.9, 8.0252) centre (-28.9, 16.6854) ccw projected
  line L32 (-38.9, 16.6854) -> (-38.9, 50.0563) projected
  arc A5 (-33.9, 58.7165) -> (-38.9, 50.0563) centre (-28.9, 50.0563) ccw projected
  line L33 (-33.9, 58.7165) -> (-5, 75.4019) projected
  arc A6 (5, 75.4019) -> (-5, 75.4019) centre (0, 66.7417) ccw projected
  line L34 (5, 75.4019) -> (33.9, 58.7165) projected
  arc A7 (38.9, 50.0563) -> (33.9, 58.7165) centre (28.9, 50.0563) ccw projected
  line L35 (38.9, 50.0563) -> (38.9, 16.6854) projected
  line L36 (-13.8, 18.9708) -> (-13.8, 47.7708)
  line L37 (13.8, 47.7708) -> (13.8, 18.9708)
  constraints: 4 end point, 1 parallel, 1 vertical
extrude "Extrusion20" add sketch "Sketch22" along normal blind 5 contours L0 L1 L2 L3 | L4 L5 L6 L7 | L29 L28 L36 L12 L11 L10 L9 L8 | L27 L26 A1 L25 L24 L37 L16 L15 A0 L14 L13 L36 | L23 L22 L21 L20 L19 L18 L17 L37 | L30 A3 L31 A4 L32 A5 L33 A6 L34 A7 L35 A2 bodies 3
sketch "Sketch25" plane through (0, 0, 0) normal (0, 0, 1) x (1, 0, 0)
  line L0 (0, 30.4) -> (0, 0) projected
  line L1 (0, 0) -> (-18.7, 0) projected
  line L2 (-18.7, 0) -> (-18.7, 30.4) projected
  line L3 (-18.7, 30.4) -> (0, 30.4) projected
  line L4 (48.7, 0) -> (30, 0) projected
  line L5 (30, 0) -> (30, 30.4) projected
  line L6 (30, 30.4) -> (48.7, 30.4) projected
  line L7 (48.7, 30.4) -> (48.7, 0) projected
  line L8 (0.2, 30.6) -> (-18.9, 30.6) projected
  line L9 (-18.9, 30.6) -> (-18.9, -0.2) projected
  line L10 (-18.9, -0.2) -> (0.2, -0.2) projected
  line L11 (0.2, -0.2) -> (0.2, 0.8) projected
  line L12 (0.2, 0.8) -> (1.2, 0.8) projected
  line L13 (1.2, 0.8) -> (-4.8205, -12.501) projected
  line L14 (12.5, -22.501) -> (-4.8205, -12.501) projected
  arc A0 (12.5, -22.501) -> (17.5, -22.501) centre (15, -18.1708) ccw projected
  line L15 (34.8205, -12.501) -> (17.5, -22.501) projected
  line L16 (34.8205, -12.501) -> (28.8, 0.8) projected
  line L17 (28.8, 0.8) -> (29.8, 0.8) projected
  line L18 (29.8, 0.8) -> (29.8, -0.2) projected
  line L19 (29.8, -0.2) -> (48.9, -0.2) projected
  line L20 (48.9, 30.6) -> (48.9, -0.2) projected
  line L21 (48.9, 30.6) -> (29.8, 30.6) projected
  line L22 (29.8, 30.6) -> (29.8, 29.6) projected
  line L23 (29.8, 29.6) -> (28.8, 29.6) projected
  line L24 (28.8, 29.6) -> (34.8205, 42.901) projected
  line L25 (17.5, 52.901) -> (34.8205, 42.901) projected
  arc A1 (17.5, 52.901) -> (12.5, 52.901) centre (15, 48.5708) ccw projected
  line L26 (-4.8205, 42.901) -> (12.5, 52.901) projected
  line L27 (-4.8205, 42.901) -> (1.2, 29.6) projected
  line L28 (1.2, 29.6) -> (0.2, 29.6) projected
  line L29 (0.2, 29.6) -> (0.2, 30.6) projected
  line L30 (-18.9, 40.5457) -> (10, 57.2311) projected
  arc A2 (20, 57.2311) -> (10, 57.2311) centre (15, 48.5708) ccw projected
  line L31 (20, 57.2311) -> (48.9, 40.5457) projected
  arc A3 (53.9, 31.8854) -> (48.9, 40.5457) centre (43.9, 31.8854) ccw projected
  line L32 (53.9, 31.8854) -> (53.9, -1.4854) projected
  arc A4 (48.9, -10.1457) -> (53.9, -1.4854) centre (43.9, -1.4854) ccw projected
  line L33 (48.9, -10.1457) -> (20, -26.8311) projected
  arc A5 (10, -26.8311) -> (20, -26.8311) centre (15, -18.1708) ccw projected
  line L34 (10, -26.8311) -> (-18.9, -10.1457) projected
  arc A6 (-23.9, -1.4854) -> (-18.9, -10.1457) centre (-13.9, -1.4854) ccw projected
  line L35 (-23.9, -1.4854) -> (-23.9, 31.8854) projected
  arc A7 (-18.9, 40.5457) -> (-23.9, 31.8854) centre (-13.9, 31.8854) ccw projected
  circle A8 centre (-10.0746, -7.1806) radius 6.9806
  circle A9 centre (-10.0746, 37.5806) radius 6.9806
  circle A10 centre (40.0746, 37.5806) radius 6.9806
  circle A11 centre (40.0746, -7.1806) radius 6.9806
  circle A12 centre (-10.0746, -7.1806) radius 1.5
  circle A13 centre (-10.0746, 37.5806) radius 1.5
  circle A14 centre (40.0746, 37.5806) radius 1.5
  circle A15 centre (40.0746, -7.1806) radius 1.5
  dimension "d135" = 3
  dimension "d136" = 3
  dimension "d137" = 3
  dimension "d138" = 3
  constraints: 12 tangent, 8 centre point, 4 coincident
  measures "d135" diameter of A12
  measures "d136" diameter of A13
  measures "d137" diameter of A14
  measures "d138" diameter of A15
extrude "Extrusion21" cut sketch "Sketch25" along normal through all both and the other way through all contours A12 | A13 | A14 | A15 bodies 2 3
sketch "Sketch26" plane through (15, -18.1708, 13.5) normal (0, 0, 1) x (1, 0, 0)
  circle A0 centre (25.0746, 55.7514) radius 1.5 projected
  circle A1 centre (25.0746, 10.9903) radius 1.5 projected
  circle A2 centre (-25.0746, 55.7514) radius 1.5 projected
  circle A3 centre (-25.0746, 10.9903) radius 1.5 projected
  line L0 (33.9, 8.0252) -> (5, -8.6603) projected
  arc A4 (-5, -8.6603) -> (5, -8.6603) centre (0, 0) ccw projected
  line L1 (-5, -8.6603) -> (-33.9, 8.0252) projected
  arc A5 (-38.9, 16.6854) -> (-33.9, 8.0252) centre (-28.9, 16.6854) ccw projected
  line L2 (-38.9, 16.6854) -> (-38.9, 50.0563) projected
  arc A6 (-33.9, 58.7165) -> (-38.9, 50.0563) centre (-28.9, 50.0563) ccw projected
  line L3 (-33.9, 58.7165) -> (-5, 75.4019) projected
  arc A7 (5, 75.4019) -> (-5, 75.4019) centre (0, 66.7417) ccw projected
  line L4 (5, 75.4019) -> (33.9, 58.7165) projected
  arc A8 (38.9, 50.0563) -> (33.9, 58.7165) centre (28.9, 50.0563) ccw projected
  line L5 (38.9, 50.0563) -> (38.9, 16.6854) projected
  arc A9 (33.9, 8.0252) -> (38.9, 16.6854) centre (28.9, 16.6854) ccw projected
  circle A10 centre (-25.0746, 10.9903) radius 2.9
  circle A11 centre (-25.0746, 55.7514) radius 1.5 projected
  circle A12 centre (-25.0746, 55.7514) radius 2.9
  circle A13 centre (25.0746, 55.7514) radius 2.9
  circle A14 centre (25.0746, 10.9903) radius 2.9
  point P0 (-15, 18.1708)
  dimension "d141" = 5.8
  dimension "d142" = 5.8
  dimension "d143" = 5.8
  dimension "d144" = 5.8
  constraints: 4 centre point, 4 coincident
  measures "d141" diameter of A10
  measures "d142" diameter of A12
  measures "d143" diameter of A14
  measures "d144" diameter of A13
extrude "Extrusion22" cut sketch "Sketch26" against normal blind 3 contours A0 | A3 | A10 | A12 | A13 | A14 bodies 3
sketch "Sketch27" plane through (0, 0, -5) normal (0, 0, -1) x (-1, 0, 0)
  circle A0 centre (-40.0746, 37.5806) radius 1.5 projected
  circle A1 centre (-40.0746, -7.1806) radius 1.5 projected
  circle A2 centre (10.0746, 37.5806) radius 1.5 projected
  circle A3 centre (10.0746, -7.1806) radius 1.5 projected
  line L0 (-10, 57.2311) -> (18.9, 40.5457) projected
  arc A4 (23.9, 31.8854) -> (18.9, 40.5457) centre (13.9, 31.8854) ccw projected
  line L1 (23.9, 31.8854) -> (23.9, -1.4854) projected
  arc A5 (18.9, -10.1457) -> (23.9, -1.4854) centre (13.9, -1.4854) ccw projected
  line L2 (18.9, -10.1457) -> (-10, -26.8311) projected
  arc A6 (-20, -26.8311) -> (-10, -26.8311) centre (-15, -18.1708) ccw projected
  line L3 (-20, -26.8311) -> (-48.9, -10.1457) projected
  arc A7 (-53.9, -1.4854) -> (-48.9, -10.1457) centre (-43.9, -1.4854) ccw projected
  line L4 (-53.9, -1.4854) -> (-53.9, 31.8854) projected
  arc A8 (-48.9, 40.5457) -> (-53.9, 31.8854) centre (-43.9, 31.8854) ccw projected
  line L5 (-48.9, 40.5457) -> (-20, 57.2311) projected
  arc A9 (-10, 57.2311) -> (-20, 57.2311) centre (-15, 48.5708) ccw projected
  circle A10 centre (-40.0746, -7.1806) radius 2.9 projected
  circle A11 centre (-40.0746, -7.1806) radius 2.1
  circle A12 centre (-40.0746, 37.5806) radius 2.9 projected
  circle A13 centre (-40.0746, 37.5806) radius 2.1
  circle A14 centre (10.0746, -7.1806) radius 2.9 projected
  circle A15 centre (10.0746, -7.1806) radius 2.1
  circle A16 centre (10.0746, 37.5806) radius 2.9 projected
  circle A17 centre (10.0746, 37.5806) radius 2.1
  point P0 (0, 0)
  dimension "d147" = 4.2
  dimension "d148" = 4.2
  dimension "d149" = 4.2
  dimension "d150" = 4.2
  constraints: 4 centre point, 4 coincident
  measures "d147" diameter of A11
  measures "d148" diameter of A13
  measures "d149" diameter of A15
  measures "d150" diameter of A17
extrude "Extrusion23" cut sketch "Sketch27" against normal blind 6 contours A0 | A1 | A2 | A3 | A10 | A11 | A12 | A13 | A14 | A15 | A16 | A17 bodies 2
chamfer "Chamfer1" distance 1 angle 45 8 edges at (42.9746, -7.1806, -5) (42.9746, 37.5806, -5) (-7.1746, 37.5806, -5) (-7.1746, -7.1806, -5) (-12.9746, 37.5806, 13.5) (37.1746, 37.5806, 13.5) (37.1746, -7.1806, 13.5) (-12.9746, -7.1806, 13.5)
fillet "Fillet3" radius 3 24 edges at (-22.5603, -6.4854, -5) (-23.9, 15.2, -5) (-22.5603, 36.8854, -5) (-4.45, 48.8884, -5) (15, 58.5708, -5) (34.45, 48.8884, -5) (52.5603, 36.8854, -5) (53.9, 15.2, -5) (52.5603, -6.4854, -5) (34.45, -18.4884, -5) (15, -28.1708, -5) (-4.45, -18.4884, -5) (15, -28.1708, 13.5) (34.45, -18.4884, 13.5) (52.5603, -6.4854, 13.5) (53.9, 15.2, 13.5) (52.5603, 36.8854, 13.5) (34.45, 48.8884, 13.5) (15, 58.5708, 13.5) (-4.45, 48.8884, 13.5) (-22.5603, 36.8854, 13.5) (-23.9, 15.2, 13.5) (-22.5603, -6.4854, 13.5) (-4.45, -18.4884, 13.5)
ref_plane "Work Plane10" through (0.2, 15.2, 3.25) normal (0, -1, 0) x (1, 0, 0)
mirror "Mirror6" about plane through (0.2, 15.2, 3.25) normal (0, -1, 0) of "Extrusion16", "Mirror5" bodies 2 3
sketch "Sketch28" plane through (15, -18.1708, 13.5) normal (0, 0, 1) x (1, 0, 0)
  line L0 (-22.5, 41.1208) -> (22.5, 41.1208) construction
  line L1 (22.5, 41.1208) -> (22.5, 25.6208) construction
  line L2 (22.5, 25.6208) -> (-22.5, 25.6208) construction
  line L3 (-22.5, 25.6208) -> (-22.5, 41.1208) construction
  arc A0 (-3.5, -6.0622) -> (3.5, -6.0622) centre (0, 0) ccw projected
  line L4 (3.5, -6.0622) -> (32.4, 10.6232) projected
  arc A1 (32.4, 10.6232) -> (35.9, 16.6854) centre (28.9, 16.6854) ccw projected
  line L5 (35.9, 16.6854) -> (35.9, 50.0563) projected
  arc A2 (35.9, 50.0563) -> (32.4, 56.1184) centre (28.9, 50.0563) ccw projected
  line L6 (32.4, 56.1184) -> (3.5, 72.8039) projected
  arc A3 (3.5, 72.8039) -> (-3.5, 72.8039) centre (0, 66.7417) ccw projected
  line L7 (-3.5, 72.8039) -> (-32.4, 56.1184) projected
  arc A4 (-32.4, 56.1184) -> (-35.9, 50.0563) centre (-28.9, 50.0563) ccw projected
  line L8 (-35.9, 50.0563) -> (-35.9, 16.6854) projected
  arc A5 (-35.9, 16.6854) -> (-32.4, 10.6232) centre (-28.9, 16.6854) ccw projected
  line L9 (-32.4, 10.6232) -> (-3.5, -6.0622) projected
  circle A6 centre (-25.0746, 10.9903) radius 3.9 projected
  circle A7 centre (25.0746, 55.7514) radius 3.9 projected
  circle A8 centre (-25.0746, 55.7514) radius 3.9 projected
  circle A9 centre (25.0746, 10.9903) radius 3.9 projected
  line L10 (-35.9, 33.3708) -> (35.9, 33.3708)
  line L11 (35.9, 16.6854) -> (35.9, 50.0563) projected
  line L12 (0, 73.7417) -> (0, -7)
  spline S0 degree 2 poles (-15.1216, 25.586) (-16.5802, 25.586) (-19.0478, 26.5706) (-19.9473, 27.5552) knots 0 0 0 1 2 2 2
  spline S1 degree 2 poles (-19.9473, 27.5552) (-20.8468, 28.5277) (-21.8314, 31.445) (-21.8314, 33.3413) knots 0 0 0 1 2 2 2
  spline S2 degree 2 poles (-21.8314, 33.3413) (-21.8314, 35.2254) (-20.8712, 38.0212) (-19.9595, 39.0544) knots 0 0 0 1 2 2 2
  spline S3 degree 2 poles (-19.9595, 39.0544) (-19.06, 40.0633) (-16.6045, 41.1208) (-15.0851, 41.1208) knots 0 0 0 1 2 2 2
  spline S4 degree 2 poles (-15.0851, 41.1208) (-14.3314, 41.1208) (-13.0065, 40.902) (-12.4473, 40.7319) knots 0 0 0 1 2 2 2
  spline S5 degree 2 poles (-12.4473, 40.7319) (-11.9611, 40.5738) (-10.9522, 40.1241) (-10.4538, 39.8567) knots 0 0 0 1 2 2 2
  line L13 (-10.4538, 39.8567) -> (-10.4538, 37.4499)
  line L14 (-10.4538, 37.4499) -> (-10.6118, 37.4499)
  spline S6 degree 2 poles (-10.6118, 37.4499) (-10.8793, 37.693) (-11.7058, 38.3737) (-12.3015, 38.7019) knots 0 0 0 1 2 2 2
  spline S7 degree 2 poles (-12.3015, 38.7019) (-12.8728, 39.0179) (-14.222, 39.4191) (-15.0972, 39.4191) knots 0 0 0 1 2 2 2
  spline S8 degree 2 poles (-15.0972, 39.4191) (-16.0575, 39.4191) (-17.7715, 38.6289) (-18.4157, 37.8753) knots 0 0 0 1 2 2 2
  spline S9 degree 2 poles (-18.4157, 37.8753) (-19.0478, 37.1095) (-19.7528, 34.7878) (-19.7528, 33.3413) knots 0 0 0 1 2 2 2
  spline S10 degree 2 poles (-19.7528, 33.3413) (-19.7528, 31.7975) (-19.0113, 29.573) (-18.3671, 28.8072) knots 0 0 0 1 2 2 2
  spline S11 degree 2 poles (-18.3671, 28.8072) (-17.735, 28.0657) (-16.0454, 27.3121) (-15.0972, 27.3121) knots 0 0 0 1 2 2 2
  spline S12 degree 2 poles (-15.0972, 27.3121) (-14.2342, 27.3121) (-12.7634, 27.7375) (-12.1921, 28.0536) knots 0 0 0 1 2 2 2
  spline S13 degree 2 poles (-12.1921, 28.0536) (-11.6451, 28.3696) (-10.8306, 29.026) (-10.5997, 29.257) knots 0 0 0 1 2 2 2
  line L15 (-10.5997, 29.257) -> (-10.4538, 29.257)
  line L16 (-10.4538, 29.257) -> (-10.4538, 26.8745)
  spline S14 degree 2 poles (-10.4538, 26.8745) (-10.9522, 26.6435) (-11.8274, 26.2181) (-12.4473, 26.0236) knots 0 0 0 1 2 2 2
  spline S15 degree 2 poles (-12.4473, 26.0236) (-13.1037, 25.8048) (-14.222, 25.586) (-15.1216, 25.586) knots 0 0 0 1 2 2 2
  line L17 (-3.3671, 25.8534) -> (-9.1775, 25.8534)
  line L18 (-9.1775, 25.8534) -> (-9.1775, 27.385)
  line L19 (-9.1775, 27.385) -> (-7.269, 27.385)
  line L20 (-7.269, 27.385) -> (-7.269, 39.3218)
  line L21 (-7.269, 39.3218) -> (-9.1775, 39.3218)
  line L22 (-9.1775, 39.3218) -> (-9.1775, 40.8534)
  line L23 (-9.1775, 40.8534) -> (-3.3671, 40.8534)
  line L24 (-3.3671, 40.8534) -> (-3.3671, 39.3218)
  line L25 (-3.3671, 39.3218) -> (-5.2755, 39.3218)
  line L26 (-5.2755, 39.3218) -> (-5.2755, 27.385)
  line L27 (-5.2755, 27.385) -> (-3.3671, 27.385)
  line L28 (-3.3671, 27.385) -> (-3.3671, 25.8534)
  line L29 (10.7091, 25.8534) -> (8.1199, 25.8534)
  line L30 (8.1199, 25.8534) -> (3.3793, 31.8218)
  line L31 (3.3793, 31.8218) -> (1.094, 31.8218)
  line L32 (1.094, 31.8218) -> (1.094, 25.8534)
  line L33 (1.094, 25.8534) -> (-0.8995, 25.8534)
  line L34 (-0.8995, 25.8534) -> (-0.8995, 40.8534)
  line L35 (-0.8995, 40.8534) -> (2.966, 40.8534)
  spline S16 degree 2 poles (2.966, 40.8534) (4.2545, 40.8534) (5.9927, 40.5738) (6.7828, 40.0633) knots 0 0 0 1 2 2 2
  spline S17 degree 2 poles (6.7828, 40.0633) (7.5729, 39.5528) (8.4846, 37.9604) (8.4846, 36.7813) knots 0 0 0 1 2 2 2
  spline S18 degree 2 poles (8.4846, 36.7813) (8.4846, 35.1403) (6.8071, 32.9158) (5.3728, 32.381) knots 0 0 0 1 2 2 2
  line L36 (5.3728, 32.381) -> (10.7091, 25.8534)
  spline S19 degree 2 poles (6.406, 36.6233) (6.406, 37.2797) (5.9441, 38.2886) (5.4579, 38.6168) knots 0 0 0 1 2 2 2
  spline S20 degree 2 poles (5.4579, 38.6168) (5.0324, 38.8964) (3.9019, 39.1273) (3.0754, 39.1273) knots 0 0 0 1 2 2 2
  line L37 (3.0754, 39.1273) -> (1.094, 39.1273)
  line L38 (1.094, 39.1273) -> (1.094, 33.4871)
  line L39 (1.094, 33.4871) -> (2.8444, 33.4871)
  spline S21 degree 2 poles (2.8444, 33.4871) (3.7075, 33.4871) (5.081, 33.791) (5.5551, 34.2651) knots 0 0 0 1 2 2 2
  spline S22 degree 2 poles (5.5551, 34.2651) (5.9927, 34.6784) (6.406, 35.8453) (6.406, 36.6233) knots 0 0 0 1 2 2 2
  spline S23 degree 2 poles (17.7593, 25.586) (16.3006, 25.586) (13.8331, 26.5706) (12.9335, 27.5552) knots 0 0 0 1 2 2 2
  spline S24 degree 2 poles (12.9335, 27.5552) (12.034, 28.5277) (11.0494, 31.445) (11.0494, 33.3413) knots 0 0 0 1 2 2 2
  spline S25 degree 2 poles (11.0494, 33.3413) (11.0494, 35.2254) (12.0097, 38.0212) (12.9214, 39.0544) knots 0 0 0 1 2 2 2
  spline S26 degree 2 poles (12.9214, 39.0544) (13.8209, 40.0633) (16.2763, 41.1208) (17.7958, 41.1208) knots 0 0 0 1 2 2 2
  spline S27 degree 2 poles (17.7958, 41.1208) (18.5494, 41.1208) (19.8744, 40.902) (20.4335, 40.7319) knots 0 0 0 1 2 2 2
  spline S28 degree 2 poles (20.4335, 40.7319) (20.9198, 40.5738) (21.9287, 40.1241) (22.4271, 39.8567) knots 0 0 0 1 2 2 2
  line L40 (22.4271, 39.8567) -> (22.4271, 37.4499)
  line L41 (22.4271, 37.4499) -> (22.269, 37.4499)
  spline S29 degree 2 poles (22.269, 37.4499) (22.0016, 37.693) (21.175, 38.3737) (20.5794, 38.7019) knots 0 0 0 1 2 2 2
  spline S30 degree 2 poles (20.5794, 38.7019) (20.0081, 39.0179) (18.6588, 39.4191) (17.7836, 39.4191) knots 0 0 0 1 2 2 2
  spline S31 degree 2 poles (17.7836, 39.4191) (16.8233, 39.4191) (15.1094, 38.6289) (14.4652, 37.8753) knots 0 0 0 1 2 2 2
  spline S32 degree 2 poles (14.4652, 37.8753) (13.8331, 37.1095) (13.128, 34.7878) (13.128, 33.3413) knots 0 0 0 1 2 2 2
  spline S33 degree 2 poles (13.128, 33.3413) (13.128, 31.7975) (13.8695, 29.573) (14.5138, 28.8072) knots 0 0 0 1 2 2 2
  spline S34 degree 2 poles (14.5138, 28.8072) (15.1459, 28.0657) (16.8355, 27.3121) (17.7836, 27.3121) knots 0 0 0 1 2 2 2
  spline S35 degree 2 poles (17.7836, 27.3121) (18.6467, 27.3121) (20.1175, 27.7375) (20.6888, 28.0536) knots 0 0 0 1 2 2 2
  spline S36 degree 2 poles (20.6888, 28.0536) (21.2358, 28.3696) (22.0502, 29.026) (22.2812, 29.257) knots 0 0 0 1 2 2 2
  line L42 (22.2812, 29.257) -> (22.4271, 29.257)
  line L43 (22.4271, 29.257) -> (22.4271, 26.8745)
  spline S37 degree 2 poles (22.4271, 26.8745) (21.9287, 26.6435) (21.0535, 26.2181) (20.4335, 26.0236) knots 0 0 0 1 2 2 2
  spline S38 degree 2 poles (20.4335, 26.0236) (19.7771, 25.8048) (18.6588, 25.586) (17.7593, 25.586) knots 0 0 0 1 2 2 2
  point P0 (-15, 18.1708)
  point P1 (-22.5, 33.3708)
  point P2 (0, 41.1208)
  dimension "d157" = 15.5
  dimension "d158" = 45
  dimension "d159" = 0
  dimension "d160" = 0
  constraints: 4 end point, 4 midpoint, 2 point on circle, 1 parallel, 2 other
  measures "d157" distance between parallel lines of L2 L0
  measures "d158" distance between parallel lines of L1 L3
  measures "d159" distance from line of L10 point (-22.5, 33.371)
  measures "d160" distance from line of L12 point (0, 41.121)